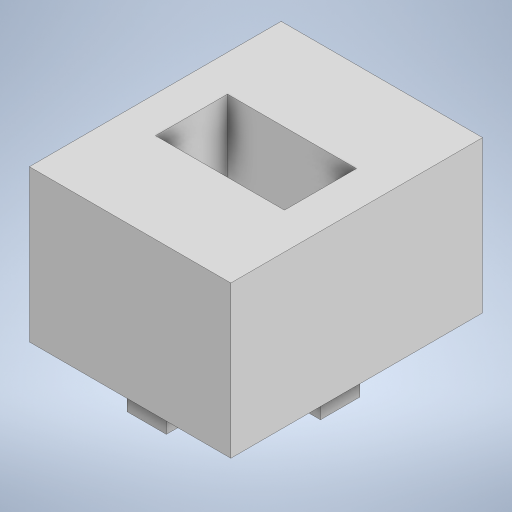
# Autodesk Inventor part: magnet_jig
Saved by Autodesk Inventor 2023 (Build 270158000, 158)
## iProperties
Created: 2023-04-11
Part Number: magnet_jig
Material: Generic
Document SubType Name: Modeling
Designer: Sam
Density: 1 g/cm^3
Appearance: Default
Author: Sam
Autodesk Inventor part; units mm, degrees
ref_plane "YZ Plane" through (0, 0, 0) normal (1, 0, 0) x (0, 1, 0)
ref_plane "XZ Plane" through (0, 0, 0) normal (0, 1, 0) x (-1, 0, 0)
ref_plane "XY Plane" through (0, 0, 0) normal (0, 0, 1) x (1, 0, 0)
sketch "Sketch1" plane through (0, 0, 0) normal (0, 1, 0) x (-1, 0, 0)
  line L0 (-8.128, 10.16) -> (8.128, 10.16)
  line L1 (8.128, 10.16) -> (8.128, -10.16)
  line L2 (8.128, -10.16) -> (-8.128, -10.16)
  line L3 (-8.128, -10.16) -> (-8.128, 10.16)
  line L4 (-8.128, 10.16) -> (8.128, -10.16) construction
  line L5 (8.128, 10.16) -> (-8.128, -10.16) construction
  point P0 (0, 0)
  dimension "d0" = 20.32
  dimension "d1" = 16.256
  constraints: 12 end point, 2 midpoint, 2 parallel, 1 horizontal, 1 perpendicular
  measures "d0" distance of L0.end L1.end
  measures "d1" distance of L0.start L0.end
extrude "Extrusion1" add sketch "Sketch1" along normal mid plane 12.2492
sketch "Sketch3" plane through (0, -6.1246, 0) normal (0, -1, 0) x (1, 0, 0)
  line L0 (-5.203, 2.905) -> (5.203, 2.905)
  line L1 (5.203, 2.905) -> (5.203, -2.905)
  line L2 (5.203, -2.905) -> (-5.203, -2.905)
  line L3 (-5.203, -2.905) -> (-5.203, 2.905)
  line L4 (-5.203, 2.905) -> (5.203, -2.905) construction
  line L5 (5.203, 2.905) -> (-5.203, -2.905) construction
  point P0 (0, 0)
  dimension "d4" = 5.81
  dimension "d5" = 10.406
  constraints: 12 end point, 2 midpoint, 2 parallel, 1 horizontal, 1 perpendicular
  measures "d4" distance of L0.end L1.end
  measures "d5" distance of L1.end L2.end
extrude "Extrusion2" cut sketch "Sketch3" against normal through all
sketch "Sketch4" plane through (0, -6.1246, 0) normal (0, -1, 0) x (1, 0, 0)
  line L0 (-4.9149, 6.985) -> (4.9149, 6.985) construction
  line L1 (4.9149, 6.985) -> (4.9149, 4.1402) construction
  line L2 (4.9149, 4.1402) -> (-4.9149, 4.1402) construction
  line L3 (-4.9149, 4.1402) -> (-4.9149, 6.985) construction
  line L4 (-4.9149, 6.985) -> (4.9149, 4.1402) construction
  line L5 (4.9149, 6.985) -> (-4.9149, 4.1402) construction
  line L6 (5.1649, 7.235) -> (-5.1649, 7.235)
  line L7 (-5.1649, 7.235) -> (-5.1649, 3.8902)
  line L8 (-5.1649, 3.8902) -> (5.1649, 3.8902)
  line L9 (5.1649, 3.8902) -> (5.1649, 7.235)
  point P0 (0, 0)
  point P1 (0, 5.5626)
  dimension "d8" = 2.8448
  dimension "d9" = 9.8298
  dimension "d10" = 6.985
  dimension "d13" = 0.25
  constraints: 20 end point, 4 parallel, 2 midpoint, 2 perpendicular, 1 horizontal, 1 vertical alignment, 3 other
  measures "d8" distance of L0.end L1.end
  measures "d9" distance of L1.end L2.end
  measures "d10" distance from line of point (0, 0) L0
  measures "d13" distance between parallel lines of L6 L0
extrude "Extrusion3" cut sketch "Sketch4" against normal blind 2.6099
mirror "Mirror1" about plane through (0, 0, 0) normal (0, 0, 1) of "Extrusion3"
sketch "Sketch5" plane through (0, -6.1246, 0) normal (0, -1, 0) x (1, 0, 0)
  line L0 (-5.203, -2.905) -> (-5.203, 2.905) projected
  line L1 (-5.203, 1.5875) -> (-6.7905, 1.5875)
  line L2 (-6.7905, 1.5875) -> (-6.7905, -1.5875)
  line L3 (-6.7905, -1.5875) -> (-5.203, -1.5875)
  line L4 (-5.203, -1.5875) -> (-5.203, 1.5875)
  point P0 (0, 0)
  point P1 (-6.7905, 0)
  dimension "d14" = 1.5875
  dimension "d15" = 3.175
  constraints: 8 end point, 2 parallel, 1 horizontal, 1 horizontal alignment, 1 midpoint, 1 perpendicular, 1 point on line
  measures "d14" distance of L2.end L3.end
  measures "d15" distance of L1.end L2.end
extrude "Extrusion4" add sketch "Sketch5" along normal blind 2.2669
mirror "Mirror2" about plane through (0, 0, 0) normal (1, 0, 0) of "Extrusion4"
sketch "Sketch6" plane through (0, -6.1246, 0) normal (0, -1, 0) x (1, 0, 0)
  line L0 (-5.1649, 7.235) -> (5.1649, 7.235) projected
  line L1 (1.5875, 7.235) -> (-1.5875, 7.235)
  line L2 (-1.5875, 7.235) -> (-1.5875, 8.8225)
  line L3 (-1.5875, 8.8225) -> (1.5875, 8.8225)
  line L4 (1.5875, 8.8225) -> (1.5875, 7.235)
  point P0 (0, 0)
  point P1 (0, 7.235)
  dimension "d18" = 1.5875
  dimension "d19" = 3.175
  constraints: 8 end point, 2 parallel, 1 horizontal, 1 midpoint, 1 perpendicular, 1 point on line, 1 vertical alignment
  measures "d18" distance of L3.end L1.start
  measures "d19" distance of L2.end L3.end
extrude "Extrusion5" add sketch "Sketch6" along normal up to surface (2.2669 mm away)
mirror "Mirror3" about plane through (0, 0, 0) normal (0, 0, 1) of "Extrusion5"
sketch "Sketch7" plane through (0, -6.1246, 0) normal (0, -1, 0) x (1, 0, 0)
  line L0 (5.203, -2.905) -> (5.203, 2.905) projected
  line L1 (5.203, 2.905) -> (-5.203, 2.905)
  line L2 (-5.203, 2.905) -> (-5.203, 3.159)
  line L3 (-5.203, 3.159) -> (5.203, 3.159)
  line L4 (5.203, 3.159) -> (5.203, 2.905)
  point P0 (0, 0)
  point P1 (-5.203, 3.032)
  dimension "d22" = 0.254
  constraints: 8 end point, 2 parallel, 1 horizontal, 1 midpoint, 1 perpendicular, 1 vertical alignment
  measures "d22" distance of L3.end L0.end
extrude "Extrusion6" add sketch "Sketch7" along normal blind 0.62
mirror "Mirror4" about plane through (0, 0, 0) normal (0, 0, 1) of "Extrusion6"
body "Solid1"
